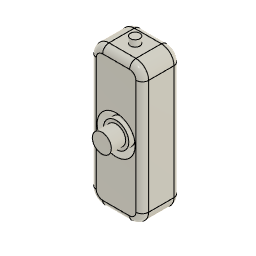
开关 v1 v2 (Autodesk Fusion 360 design; units mm, degrees)
Autodesk Fusion 360 part; units mm, degrees
sketch "草图1" plane through (0, 0, 0) normal (0, 1, 0) x (1, 0, 0)
  line L0 (4, 0) -> (12.5, 0)
  line L1 (16.5, -4) -> (16.5, -40)
  line L2 (12.5, -44) -> (4, -44)
  line L3 (0, -40) -> (0, -4)
  arc A0 (0, -40) -> (4, -44) centre (4, -40) ccw
  arc A1 (12.5, -44) -> (16.5, -40) centre (12.5, -40) ccw
  arc A2 (16.5, -4) -> (12.5, 0) centre (12.5, -4) ccw
  arc A3 (4, 0) -> (0, -4) centre (4, -4) ccw
  point P0 (16.5, 0)
  point P1 (0, -44)
  dimension "d3" = 4
  dimension "d4" = 4
  dimension "d5" = 4
  dimension "d6" = 4
  dimension "d8" = 44
  dimension "d9" = 16.5
  constraint horizontal L0
  constraint vertical L1
  constraint horizontal L2
  constraint vertical L3
  constraint coincident P1 L2
  constraint coincident P1 L3
  constraint tangent L2 A0
  constraint tangent L3 A0
  constraint tangent L2 A1
  constraint tangent L1 A1
  constraint coincident P0 L1
  constraint coincident P0 L0
  constraint tangent L1 A2
  constraint tangent L0 A2
  constraint coincident origin L3
  constraint coincident origin L0
  constraint tangent L3 A3
  constraint tangent L0 A3
  measures "d3" radius of A0
  measures "d4" radius of A1
  measures "d5" radius of A2
  measures "d6" radius of A3
  measures "d8" distance of L0 L2
  measures "d9" distance of L1 L3
extrude "拉伸1" add sketch "草图1" along normal blind 12 makes body 1
fillet "圆角1" radius 2 8 edges at (16.5, 12, 22) (15.3284, 12, 1.1716) (8.25, 12, 0) (1.1716, 12, 1.1716) (0, 12, 22) (1.1716, 12, 42.8284) (8.25, 12, 44) (15.3284, 12, 42.8284) on bodies 1
fillet "圆角2" radius 2 8 edges at (1.1716, 0, 42.8284) (0, 0, 22) (1.1716, 0, 1.1716) (8.25, 0, 0) (15.3284, 0, 1.1716) (16.5, 0, 22) (15.3284, 0, 42.8284) (8.25, 0, 44) on bodies 1
sketch "草图2" plane through (0, 0, 0) normal (0, -1, 0) x (1, 0, 0)
  arc A0 (4, 42) -> (2, 40) centre (4, 40) ccw
  line L0 (2, 40) -> (2, 4)
  arc A1 (2, 4) -> (4, 2) centre (4, 4) ccw
  line L1 (4, 2) -> (12.5, 2)
  arc A2 (12.5, 2) -> (14.5, 4) centre (12.5, 4) ccw
  line L2 (14.5, 4) -> (14.5, 40)
  arc A3 (14.5, 40) -> (12.5, 42) centre (12.5, 40) ccw
  line L3 (12.5, 42) -> (4, 42)
  circle A4 centre (8.25, 22) radius 5
  dimension "d16" = 10
  dimension "d17" = 6.25
  dimension "d18" = 20
  measures "d16" diameter of A4
  measures "d17" distance of L0 A4.centre
  measures "d18" distance of L1 A4.centre
extrude "拉伸2" cut sketch "草图2" against normal blind 2 contours A4 bodies 1
chamfer "倒角1" distance 1 angle 45 1 faces at (13.2438, 1.3333, 21.7508) on bodies 1
sketch "草图3" plane through (0, 2, 0) normal (0, -1, 0) x (1, 0, 0)
  circle A0 centre (8.25, 22) radius 4
  circle A1 centre (8.25, 22) radius 4
  circle A2 centre (8.25, 22) radius 3
  dimension "d22" = 6
  constraint concentric A0 A1
  constraint concentric A0 A2
  measures "d22" diameter of A2
extrude "拉伸3" add sketch "草图3" along normal blind 2 bodies 1
extrude "拉伸4" add 1 faces at (8.1295, 2, 22.9927) along direction (0, -1, 0) blind 6.5 on bodies 1 bodies 1
sketch "草图4" plane through (0, 0, 0) normal (0, 0, -1) x (1, 0, 0)
  line L0 (12.5, -2) -> (4, -2)
  line L1 (4, -2) -> (4, -10)
  line L2 (4, -10) -> (12.5, -10)
  line L3 (12.5, -10) -> (12.5, -2)
  circle A0 centre (8.25, -6) radius 1.5
  dimension "d27" = 3
  dimension "d29" = 4.25
  dimension "d30" = 4
  measures "d27" diameter of A0
  measures "d29" distance of L3 A0.centre
  measures "d30" distance of L2 A0.centre
extrude "拉伸5" add sketch "草图4" along normal blind 2 contours A0 bodies 1
sketch "草图5" plane through (0, 0, 44) normal (0, 0, 1) x (-1, 0, 0)
  line L0 (-4, -2) -> (-12.5, -2)
  line L1 (-12.5, -2) -> (-12.5, -10)
  line L2 (-12.5, -10) -> (-4, -10)
  line L3 (-4, -10) -> (-4, -2)
  circle A0 centre (-8.25, -6) radius 1.5
  dimension "d33" = 3
  dimension "d34" = 4
  dimension "d35" = 4.25
  measures "d33" diameter of A0
  measures "d34" distance of L0 A0.centre
  measures "d35" distance of L1 A0.centre
extrude "拉伸6" add sketch "草图5" along normal blind 2 contours A0 bodies 1
copy_body "实体->零部件1" bodies 1 removing the originals makes body 2 in component "开关"
component "开关" placed x (1, 0, 0) y (0, 1, 0) z (0, 0, 1) at (0, 0, 0)
